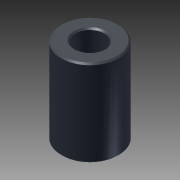
# Autodesk Inventor part: D-043
Saved by Autodesk Inventor 2015 (Build 190159000, 159)
## iProperties
Company: MARCHA TECHNOLOGY
Created: 2013-10-23
Part Number: D-043
Project: WITBOXprinter_K01
Description: CASQUILLO HOT-END
Document SubType Name: Modeling
Designer: O.Martin
Stock Number: 28655
Density: 1 g/cm^3
Material: Generic
Appearance: Dark Gray
Author: O.Martin
Autodesk Inventor part; units mm, degrees
ref_plane "YZ Plane" through (0, 0, 0) normal (1, 0, 0) x (0, 1, 0)
ref_plane "XZ Plane" through (0, 0, 0) normal (0, 1, 0) x (-1, 0, 0)
ref_plane "XY Plane" through (0, 0, 0) normal (0, 0, 1) x (1, 0, 0)
sketch "Boceto1" plane through (0, 0, 0) normal (0, 0, 1) x (1, 0, 0)
  circle A0 centre (0, 0) radius 2
  circle A1 centre (0, 0) radius 1
  dimension "d0" = 4
  dimension "d1" = 2
  constraints: 2 centre point, 2 coincident
  measures "d0" diameter of A0
  measures "d1" diameter of A1
extrude "Extrusión1" add sketch "Boceto1" along normal blind 6
chamfer "Chaflán1" distance 0.1 angle 45 4 edges at (-2, 0, 0) (-2, 0, 6) (-1, 0, 0) (-1, 0, 6)
body "Solid1"
